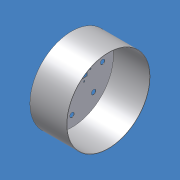
# Autodesk Inventor part: top cap
Saved by Autodesk Inventor 2015 (Build 190159000, 159)
## iProperties
Created: 2005-07-05
Part Number: top cap
Document SubType Name: Modeling
Designer: jony
Material: Generic
Density: 1 g/cm^3
Appearance: Default
Author: jony
Autodesk Inventor part; units mm, degrees
ref_plane "YZ Plane" through (0, 0, 0) normal (1, 0, 0) x (0, 1, 0)
ref_plane "XZ Plane" through (0, 0, 0) normal (0, 1, 0) x (-1, 0, 0)
ref_plane "XY Plane" through (0, 0, 0) normal (0, 0, 1) x (1, 0, 0)
sketch "Sketch1" plane through (0, 0, 0) normal (1, 0, 0) x (0, 1, 0)
  circle A0 centre (0, 0) radius 86.5188
  circle A1 centre (0, 63.5) radius 4.7625
  circle A2 centre (-44.9013, 44.9013) radius 4.7625
  circle A3 centre (-63.5, 0) radius 4.7625
  circle A4 centre (-44.9013, -44.9013) radius 4.7625
  circle A5 centre (0, -63.5) radius 4.7625
  circle A6 centre (44.9013, -44.9013) radius 4.7625
  circle A7 centre (63.5, 0) radius 4.7625
  circle A8 centre (44.9013, 44.9013) radius 4.7625
  line L0 (-31.75, 9.525) -> (31.75, 9.525)
  line L1 (31.75, 9.525) -> (31.75, -9.525)
  line L2 (31.75, -9.525) -> (-31.75, -9.525)
  line L3 (-31.75, -9.525) -> (-31.75, 9.525)
  circle A9 centre (0, 15.875) radius 1.5875
  circle A10 centre (-25.4, 15.875) radius 1.5875
  circle A11 centre (25.4, 15.875) radius 1.5875
  circle A12 centre (0, -15.875) radius 1.5875
  circle A13 centre (-25.4, -15.875) radius 1.5875
  circle A14 centre (25.4, -15.875) radius 1.5875
  circle A15 centre (-38.1, 0) radius 1.5875
  circle A16 centre (38.1, 0) radius 1.5875
  point P0 (0, 9.525)
  point P1 (-31.75, 0)
  dimension "d0" = 173.0375
  dimension "d3" = 360
  dimension "d5" = 9.525
  dimension "d6" = 63.5
  dimension "d7" = 63.5
  dimension "d8" = 19.05
  dimension "d9" = 3.175
  dimension "d10" = 15.875
  dimension "d13" = 25.4
  dimension "d20" = 25.4
  dimension "d27" = 31.75
  dimension "d32" = 38.1
  dimension "d33" = 3.175
  dimension "d36" = 76.2
  constraints: 17 centre point, 8 end point, 4 horizontal, 3 vertical alignment, 2 horizontal alignment, 2 midpoint, 2 parallel, 1 coincident, 1 perpendicular, 1 vertical, 29 other
  measures "d0" diameter of A0
  measures "d5" diameter of A8
  measures "d6" distance of A8.centre point (0, 0)
  measures "d7" distance of L0.start L0.end
  measures "d8" distance of L2.end L0.start
  measures "d9" diameter of A9
  measures "d10" distance of point (0, 0) A9.centre
  measures "d13" distance of A9.centre A10.centre
  measures "d20" distance of A9.centre A11.centre
  measures "d27" distance of A10.centre A13.centre
  measures "d32" distance of A15.centre point (0, 0)
  measures "d33" diameter of A15
  measures "d36" distance of A15.centre A16.centre
extrude "Extrusion1" add sketch "Sketch1" along normal blind 76.2
hole "Hole1" at (76.2, 0, 0) direction (-1, 0, 0) diameter 171.45 depth 75.4062
body "Solid1"
